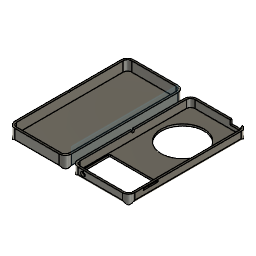
Aeropod_Case (Autodesk Fusion 360 design; units mm, degrees)
Autodesk Fusion 360 part; units mm, degrees
sketch "Sketch1" plane through (0, 0, 0) normal (0, 0, 1) x (1, 0, 0)
  line L0 (-17.51, -47.085) -> (17.51, -47.085)
  line L1 (22.51, -42.085) -> (22.51, 42.085)
  line L2 (17.51, 47.085) -> (-17.51, 47.085)
  line L3 (-22.51, 42.085) -> (-22.51, -42.085)
  arc A0 (17.51, -47.085) -> (22.51, -42.085) centre (17.51, -42.085) ccw
  arc A1 (22.51, 42.085) -> (17.51, 47.085) centre (17.51, 42.085) ccw
  arc A2 (-17.51, 47.085) -> (-22.51, 42.085) centre (-17.51, 42.085) ccw
  arc A3 (-22.51, -42.085) -> (-17.51, -47.085) centre (-17.51, -42.085) ccw
extrude "Extrude1" add sketch "Sketch1" along normal blind 17.005 makes body 1
fillet "Fillet1" radius 2.5 4 edges at (-22.51, 0, 17.005) (0, 47.085, 17.005) (22.51, 0, 17.005) (0, -47.085, 17.005) on bodies 1
fillet "Fillet2" radius 1.5 4 edges at (-22.51, 0, 0) (0, 47.085, 0) (22.51, 0, 0) (0, -47.085, 0) on bodies 1
sketch "Sketch2" plane through (0, 0, 0) normal (0, 0, 1) x (1, 0, 0)
  line L0 (-17.51, -45.585) -> (17.51, -45.585)
  line L1 (21.01, -42.085) -> (21.01, 42.085)
  line L2 (17.51, 45.585) -> (-17.51, 45.585)
  line L3 (-21.01, 42.085) -> (-21.01, -42.085)
  arc A0 (17.51, -45.585) -> (21.01, -42.085) centre (17.51, -42.085) ccw
  arc A1 (21.01, 42.085) -> (17.51, 45.585) centre (17.51, 42.085) ccw
  arc A2 (-17.51, 45.585) -> (-21.01, 42.085) centre (-17.51, 42.085) ccw
  arc A3 (-21.01, -42.085) -> (-17.51, -45.585) centre (-17.51, -42.085) ccw
extrude "Extrude2" cut sketch "Sketch2" along normal blind 15.505 bodies 1
ref_plane "WorkPlane1" through (0, 0, 17.005) normal (0, 0, 1) x (1, 0, 0)
sketch "Sketch3" plane through (0, 0, 17.005) normal (0, 0, 1) x (1, 0, 0)
  line L0 (-19.01, 1.626) -> (19.01, 1.626)
  line L1 (20.01, 2.626) -> (20.01, 42.585)
  line L2 (19.01, 43.585) -> (-19.01, 43.585)
  line L3 (-20.01, 42.585) -> (-20.01, 2.626)
  arc A0 (19.01, 1.626) -> (20.01, 2.626) centre (19.01, 2.626) ccw
  arc A1 (20.01, 42.585) -> (19.01, 43.585) centre (19.01, 42.585) ccw
  arc A2 (-19.01, 43.585) -> (-20.01, 42.585) centre (-19.01, 42.585) ccw
  arc A3 (-20.01, 2.626) -> (-19.01, 1.626) centre (-19.01, 2.626) ccw
extrude "Extrude3" cut sketch "Sketch3" against normal blind 1.7 bodies 1
sketch "Sketch4" plane through (0, 0, 17.005) normal (0, 0, 1) x (1, 0, 0)
  circle A0 centre (0, -18.234) radius 16.86
extrude "Extrude4" cut sketch "Sketch4" against normal blind 1.7 bodies 1
ref_plane "WorkPlane2" through (0, 47.085, 0) normal (0, 1, 0) x (0, 0, 1)
sketch "Sketch5" plane through (0, 47.085, 0) normal (0, 1, 0) x (1, 0, 0)
  circle A0 centre (-13.66, -12.2436) radius 1.75
extrude "Extrude5" cut sketch "Sketch5" against normal blind 2 bodies 1
sketch "Sketch6" plane through (0, 47.085, 0) normal (0, 1, 0) x (1, 0, 0)
  line L0 (8.07, -13.4936) -> (14.07, -13.4936)
  line L1 (14.07, -13.4936) -> (14.07, -10.9936)
  line L2 (14.07, -10.9936) -> (8.07, -10.9936)
  line L3 (8.07, -10.9936) -> (8.07, -13.4936)
extrude "Extrude6" cut sketch "Sketch6" against normal blind 2 bodies 1
sketch "Sketch7" plane through (0, 47.085, 0) normal (0, 1, 0) x (1, 0, 0)
  line L0 (5.63, -10.3527) -> (17.63, -10.3527)
  line L1 (17.63, -10.3527) -> (17.63, -8.3527)
  line L2 (17.63, -8.3527) -> (5.63, -8.3527)
  line L3 (5.63, -8.3527) -> (5.63, -10.3527)
extrude "Extrude7" cut sketch "Sketch7" against normal blind 2 bodies 1
ref_plane "WorkPlane3" through (0, -47.085, 0) normal (0, 1, 0) x (0, 0, 1)
sketch "Sketch8" plane through (0, -47.085, 0) normal (0, 1, 0) x (1, 0, 0)
  line L0 (10.3, -12.8032) -> (19.3, -12.8032)
  line L1 (19.3, -12.8032) -> (19.3, -9.3032)
  line L2 (19.3, -9.3032) -> (10.3, -9.3032)
  line L3 (10.3, -9.3032) -> (10.3, -12.8032)
extrude "Extrude8" cut sketch "Sketch8" along normal blind 2 bodies 1
ref_plane "WorkPlane4" through (-22.51, 0, 0) normal (1, 0, 0) x (0, 1, 0)
sketch "Sketch9" plane through (-22.51, 0, 0) normal (1, 0, 0) x (0, 0, -1)
  circle A0 centre (5.0144, 12.7537) radius 1
  circle A1 centre (-2.9174, 12.7537) radius 1
extrude "Extrude9" cut sketch "Sketch9" along normal blind 2 bodies 1
move_body "Move1" bodies 1 to x (1, 0, 0) y (0, 1, 0) z (0, 0, 1) at (70, 0, 0)
extrude "Extrude10" add 1 faces at (82.07, 46.585, 10.9936) along direction (0, 0, 1) blind 2.5 on bodies 1 bodies 1
extrude "Extrude11" add 1 faces at (79.59, 46.085, 8.3527) along direction (0, 0, 1) blind 2 on bodies 1 bodies 1
extrude "Extrude12" add 1 faces at (63.6633, 1.626, 16.505) along direction (0, 1, 0) blind 18 on bodies 1 bodies 1
extrude "Extrude13" add 1 faces at (50.99, 13.626, 16.505) along direction (-1, 0, 0) blind 1 on bodies 1 bodies 1
extrude "Extrude14" add 1 faces at (89.01, 7.626, 16.505) along direction (1, 0, 0) blind 1 on bodies 1 bodies 1
fillet "Fillet3" radius 1 tangency weight 1.40048 1 edges at (90.01, 19.626, 16.255) on bodies 1
fillet "Fillet4" radius 1 1 edges at (49.99, 19.626, 16.255) on bodies 1
sketch "Sketch10" plane through (47.49, 0, 0) normal (-1, 0, 0) x (0, -1, 0)
  circle A0 centre (-12.7537, 2.9174) radius 1
  line L0 (-42.085, 1.5) -> (42.085, 1.5)
  line L1 (42.085, 1.5) -> (42.085, 14.505)
  line L2 (42.085, 14.505) -> (-42.085, 14.505)
  line L3 (-42.085, 14.505) -> (-42.085, 1.5)
sketch "Sketch11" plane through (0, 0, 0) normal (0, 0, 1) x (1, 0, 0)
  line L0 (91.01, 45.585) -> (91.01, -45.585)
  line L1 (91.01, -45.585) -> (48.99, -45.585)
  line L2 (48.99, -45.585) -> (48.99, 45.585)
  line L3 (48.99, 45.585) -> (91.01, 45.585)
  constraint vertical L0
  constraint perpendicular L0 L1
  constraint perpendicular L1 L2
  constraint perpendicular L0 L3
extrude "Extrude15" add sketch "Sketch11" along normal blind 1 bodies 1
extrude "Extrude16" add 1 faces at (62.9967, -14.0283, 1) along direction (0, 0, 1) blind 0.5 on bodies 1 bodies 1
extrude "Extrude17" add sketch "Sketch10" against normal blind 1.5 contours A0 bodies 1
sketch "Sketch12" plane through (47.49, 0, 0) normal (-1, 0, 0) x (0, -1, 0)
  line L0 (-42.085, 1.5) -> (42.085, 1.5)
  line L1 (42.085, 1.5) -> (42.085, 14.505)
  line L2 (42.085, 14.505) -> (-42.085, 14.505)
  line L3 (-42.085, 14.505) -> (-42.085, 1.5)
  circle A0 centre (0, 10) radius 1
extrude "Extrude18" cut sketch "Sketch12" against normal blind 6 contours A0 bodies 1
sketch "Sketch13" plane through (92.51, 0, 0) normal (1, 0, 0) x (0, 1, 0)
  line L0 (-42.085, 1.5) -> (42.085, 1.5)
  line L1 (42.085, 1.5) -> (42.085, 14.505)
  line L2 (42.085, 14.505) -> (-42.085, 14.505)
  line L3 (-42.085, 14.505) -> (-42.085, 1.5)
sketch "Sketch14" plane through (92.51, 0, 0) normal (1, 0, 0) x (0, 1, 0)
  line L0 (35.25, 9.9) -> (23.75, 9.9)
  line L1 (23.75, 9.9) -> (23.75, 11.1)
  line L2 (23.75, 11.1) -> (35.25, 11.1)
  line L3 (35.25, 11.1) -> (35.25, 9.9)
  dimension "d51" = 11.5
  dimension "d52" = 1.2
  constraint horizontal L0
  constraint vertical L1
  constraint horizontal L2
  constraint vertical L3
  measures "d51" distance of L0.start L0.end
  measures "d52" distance of L0.start L2.end
extrude "Extrude19" cut sketch "Sketch14" against normal blind 10 bodies 1
split "Split1" by plane through (89.3, -47.085, 9.3032) normal (0, 0, 1) bodies 1 makes body 2 at (70.42, 12.6103, 15.505)
move_body "Move2" bodies 2 to x (1, 0, 0) y (0, -1, 0) z (0, 0, -1) at (50, 11.6549, 34.01)
move_body "Move3" bodies 2 to x (1, 0, 0) y (0, 1, 0) z (0, 0, 1) at (0, 0, -16.7)
move_body "Move4" bodies 2 to x (1, 0, 0) y (0, 1, 0) z (0, 0, 1) at (0, 0, -0.3)
move_body "Move5" bodies 2 to x (1, 0, 0) y (0, 1, 0) z (0, 0, 1) at (0, -11.6, 0)
equation "d10 = -( 1.70 mm )"
equation "d12 = -( 1.70 mm )"
equation "d15 = -( 2.00 mm )"
equation "d17 = -( 2.00 mm )"
equation "d19 = -( 2.00 mm )"
named bodies: "Case_Body", "Case_Body (1)"
